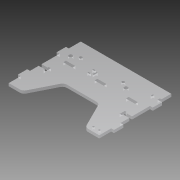
# Autodesk Inventor part: plastic_part_1
Saved by Autodesk Inventor 2013 (Build 170138000, 138)
## iProperties
Shininess: 20.0
Created: 2013-02-12
Part Number: plastic_part_1
Document SubType Name: Modeling
Designer: Noa Izumi
Material: Default
Density: 1 g/cm^3
Density: 0.0
Volumn: 0.0
Area: 0.0
PropertySet Name: Model Information
Control State: 0
Master: False
Checked Out: False
Author: Noa Izumi
Autodesk Inventor part; units mm, degrees
ref_plane "YZ Plane" through (0, 0, 0) normal (1, 0, 0) x (0, 1, 0)
ref_plane "XZ Plane" through (0, 0, 0) normal (0, 1, 0) x (-1, 0, 0)
ref_plane "XY Plane" through (0, 0, 0) normal (0, 0, 1) x (1, 0, 0)
sketch "Sketch1" plane through (0, 0, 0) normal (0, 0, 1) x (1, 0, 0)
  line L0 (0, 0) -> (98, 0)
  line L1 (98, 0) -> (98, 78)
  line L2 (98, 78) -> (0, 78)
  line L3 (0, 78) -> (0, 0)
  line L4 (-3, 65) -> (101, 65)
  line L5 (101, 65) -> (101, 55)
  line L6 (101, 55) -> (-3, 55)
  line L7 (-3, 55) -> (-3, 65)
  line L8 (101, 23) -> (101, 13)
  line L9 (-3, 13) -> (-3, 23)
  line L10 (68, 30) -> (30, 30)
  line L11 (15, 0) -> (30, 30)
  line L12 (83, 0) -> (68, 30)
  line L13 (15, 0) -> (83, 0)
  line L14 (-3, 23) -> (0, 23)
  line L15 (98, 23) -> (101, 23)
  line L16 (101, 13) -> (98, 13)
  line L17 (0, 13) -> (-3, 13)
  dimension "d0" = 98
  dimension "d1" = 78
  dimension "d171" = 104
  dimension "d172" = 3
  dimension "d173" = 10
  dimension "d174" = 13
  dimension "d175" = 10
  dimension "d177" = 3
  dimension "d181" = 30
  dimension "d182" = 30
  dimension "d183" = 30
  dimension "d184" = 15
  dimension "d185" = 15
  dimension "d186" = 10
  dimension "d187" = 13
  dimension "d188" = 13
  constraints: 36 end point, 9 parallel, 6 point on line, 4 horizontal, 4 perpendicular, 1 collinear
  measures "d0" distance of L0.start L0.end
  measures "d1" distance of L2.end L0.start
  measures "d171" distance of L4.start L4.end
  measures "d172" distance between parallel lines of L3 L7
  measures "d173" distance of L6.end L4.start
  measures "d174" distance between parallel lines of L4 L2
  measures "d175" distance of L9.start L9.end
  measures "d177" distance between parallel lines of L3 L9
  measures "d181" distance from line of L10.end L3
  measures "d182" distance from line of L10.start L1
  measures "d183" distance between parallel lines of L0 L10
  measures "d184" distance of L11.start L0.start
  measures "d185" distance of L0.end L12.start
  measures "d186" distance of L8.start L8.end
  measures "d187" distance between parallel lines of L0 L16
  measures "d188" distance between parallel lines of L0 L17
extrude "Extrusion1" add sketch "Sketch1" along normal blind 3 contours L3 L6 L1 L0 L12 L10 L11 | L17 L9 L14 L3 | L6 L7 L4 L3 | L3 L4 L1 L6 | L1 L15 L8 L16 | L3 L2 L1 L4 | L1 L4 L5 L6
fillet "圓角4" radius 5 4 edges at (15, 0, 1.5) (30, 30, 1.5) (68, 30, 1.5) (83, 0, 1.5)
sketch "草圖13" plane through (0, 0, 3) normal (0, 0, 1) x (1, 0, 0)
  line L0 (98, 55) -> (98, 23) projected
  line L1 (0, 78) -> (98, 78) projected
  line L2 (0, 65) -> (0, 78) projected
  line L3 (0, 23) -> (0, 55) projected
  line L4 (10, 52) -> (20, 52)
  line L5 (20, 52) -> (20, 49)
  line L6 (20, 49) -> (10, 49)
  line L7 (10, 49) -> (10, 52)
  line L8 (44, 52) -> (54, 52)
  line L9 (54, 52) -> (54, 49)
  line L10 (54, 49) -> (44, 49)
  line L11 (44, 49) -> (44, 52)
  line L12 (78, 52) -> (88, 52)
  line L13 (88, 52) -> (88, 49)
  line L14 (88, 49) -> (78, 49)
  line L15 (78, 49) -> (78, 52)
  dimension "d190" = 10
  dimension "d191" = 10
  dimension "d192" = 3
  dimension "d193" = 26
  dimension "d194" = 10
  dimension "d195" = 10
  dimension "d196" = 10
  dimension "d198" = 44
  constraints: 24 end point, 6 parallel, 3 horizontal, 3 perpendicular, 2 point on line
  measures "d190" distance between parallel lines of L3 L7
  measures "d191" distance of L5.end L6.end
  measures "d192" distance of L6.end L4.start
  measures "d193" distance between parallel lines of L4 L1
  measures "d194" distance of L9.end L10.end
  measures "d195" distance of L13.end L14.end
  measures "d196" distance between parallel lines of L0 L13
  measures "d198" distance between parallel lines of L2 L11
extrude "擠出6" cut sketch "草圖13" against normal through all
sketch "草圖14" plane through (0, 0, 3) normal (0, 0, 1) x (1, 0, 0)
  line L0 (0, 78) -> (98, 78) projected
  line L1 (0, 65) -> (0, 78) projected
  point P0 (8, 59)
  point P1 (68, 59)
  dimension "d201" = 8
  dimension "d202" = 19
  dimension "d203" = 60
  measures "d201" distance from line of point (8, 59) L1
  measures "d202" distance from line of point (8, 59) L0
  measures "d203" distance of point (68, 59) point (8, 59)
hole "孔5" at (8, 59, 3) at (68, 59, 3) direction (0, 0, -1) diameter 4 end through all
sketch "草圖15" plane through (0, 0, 3) normal (0, 0, 1) x (1, 0, 0)
  line L0 (0, 78) -> (98, 78) projected
  line L1 (0, 65) -> (0, 78) projected
  point P0 (15, 63)
  point P1 (61, 63)
  dimension "d211" = 15
  dimension "d212" = 15
  dimension "d213" = 46
  measures "d211" distance from line of point (15, 63) L0
  measures "d212" distance from line of point (15, 63) L1
  measures "d213" distance of point (61, 63) point (15, 63)
hole "孔6" at (15, 63, 3) at (61, 63, 3) direction (0, 0, -1) diameter 3 end through all
sketch "草圖16" plane through (0, 0, 3) normal (0, 0, 1) x (1, 0, 0)
  line L0 (98, 0) -> (86.0902, 0) projected
  line L1 (98, 13) -> (98, 0) projected
  point P0 (93.25, 5)
  point P1 (86.75, 5)
  dimension "d221" = 5
  dimension "d222" = 4.75
  dimension "d223" = 6.5
  measures "d221" distance from line of L0 point (93.25, 5)
  measures "d222" distance from line of L1 point (93.25, 5)
  measures "d223" distance of point (93.25, 5) point (86.75, 5)
hole "孔7" at (93.25, 5, 3) at (86.75, 5, 3) direction (0, 0, -1) diameter 2 end through all
sketch "草圖17" plane through (0, 0, 3) normal (0, 0, 1) x (1, 0, 0)
  line L0 (98, 55) -> (98, 23) projected
  line L1 (0, 23) -> (0, 55) projected
  line L2 (11.9098, 0) -> (0, 0) projected
  line L3 (0, 35.5) -> (9, 35.5)
  line L4 (9, 35.5) -> (9, 32.5)
  line L5 (9, 32.5) -> (0, 32.5)
  line L6 (0, 32.5) -> (0, 35.5)
  line L7 (9, 36.75) -> (6.7, 36.75)
  line L8 (6.7, 36.75) -> (6.7, 31.25)
  line L9 (6.7, 31.25) -> (9, 31.25)
  line L10 (9, 31.25) -> (9, 36.75)
  line L11 (89, 35.5) -> (98, 35.5)
  line L12 (98, 35.5) -> (98, 32.5)
  line L13 (98, 32.5) -> (89, 32.5)
  line L14 (89, 32.5) -> (89, 35.5)
  line L15 (89, 36.75) -> (91.3, 36.75)
  line L16 (91.3, 36.75) -> (91.3, 31.25)
  line L17 (91.3, 31.25) -> (89, 31.25)
  line L18 (89, 31.25) -> (89, 36.75)
  dimension "d231" = 9
  dimension "d233" = 3
  dimension "d234" = 32.5
  dimension "d235" = 2.3
  dimension "d236" = 5.5
  dimension "d237" = 1.25
  dimension "d239" = 9
  dimension "d240" = 2.3
  constraints: 32 end point, 8 parallel, 4 horizontal, 4 perpendicular, 2 point on line
  measures "d231" distance of L3.start L3.end
  measures "d233" distance of L3.end L4.end
  measures "d234" distance between parallel lines of L2 L5
  measures "d235" distance of L8.end L9.end
  measures "d236" distance of L9.end L7.start
  measures "d237" distance between parallel lines of L5 L9
  measures "d239" distance of L11.start L11.end
  measures "d240" distance of L15.start L15.end
extrude "擠出7" cut sketch "草圖17" against normal through all
sketch "草圖18" plane through (0, 0, 3) normal (0, 0, 1) x (1, 0, 0)
  line L0 (0, 35.5) -> (0, 55) projected
  line L1 (10, 52) -> (20, 52) projected
  line L2 (37, 57.75) -> (38.5, 57.75)
  line L3 (38.5, 57.75) -> (38.5, 53.75)
  line L4 (38.5, 53.75) -> (37, 53.75)
  line L5 (37, 53.75) -> (37, 57.75)
  line L6 (35.25, 57.75) -> (32.75, 57.75)
  line L7 (32.75, 57.75) -> (32.75, 59.15)
  line L8 (32.75, 59.15) -> (35.25, 59.15)
  line L9 (35.25, 59.15) -> (35.25, 57.75)
  line L10 (35.25, 53.75) -> (32.75, 53.75)
  line L11 (32.75, 53.75) -> (32.75, 52.35)
  line L12 (32.75, 52.35) -> (35.25, 52.35)
  line L13 (35.25, 52.35) -> (35.25, 53.75)
  line L14 (98, 65) -> (96.3, 65)
  line L15 (96.3, 65) -> (96.3, 67.5)
  line L16 (96.3, 67.5) -> (98, 67.5)
  line L17 (98, 67.5) -> (98, 65)
  line L18 (90.125, 67.5) -> (88.725, 67.5)
  line L19 (88.725, 67.5) -> (88.725, 65)
  line L20 (88.725, 65) -> (90.125, 65)
  line L21 (90.125, 65) -> (90.125, 67.5)
  dimension "d243" = 37
  dimension "d244" = 1.75
  dimension "d245" = 4
  dimension "d246" = 1.5
  dimension "d247" = 2.5
  dimension "d248" = 1.4
  dimension "d249" = 1.75
  dimension "d250" = 1.4
  dimension "d254" = 1.7
  dimension "d255" = 2.5
  dimension "d256" = 1.4
  dimension "d257" = 6.175
  constraints: 40 end point, 10 parallel, 5 horizontal, 5 perpendicular
  measures "d243" distance between parallel lines of L0 L5
  measures "d244" distance between parallel lines of L1 L4
  measures "d245" distance of L4.end L2.start
  measures "d246" distance of L3.end L4.end
  measures "d247" distance of L6.start L6.end
  measures "d248" distance of L6.end L7.end
  measures "d249" distance between parallel lines of L5 L9
  measures "d250" distance of L10.end L11.end
  measures "d254" distance of L14.start L14.end
  measures "d255" distance of L14.end L15.end
  measures "d256" distance of L19.end L20.end
  measures "d257" distance between parallel lines of L15 L21
extrude "擠出8" cut sketch "草圖18" against normal through all
